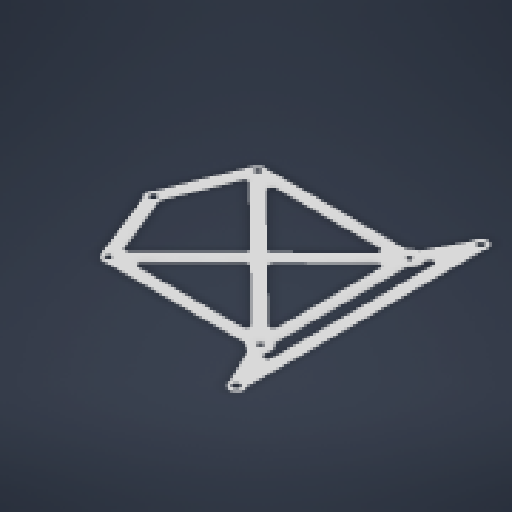
# Autodesk Inventor part: bed
Saved by Autodesk Inventor 2025 (Build 290162000, 162)
## iProperties
Created: 2024-06-24
Part Number: bed
Material: Generic
Document SubType Name: Sheet Metal
Designer: Windows 7 was better
Density: 1 g/cm^3
Sheet Metal Rule: Default_mm
Appearance: Default
Author: Windows 7 was better
Autodesk Inventor part; units mm, degrees
ref_plane "YZ Plane" through (0, 0, 0) normal (1, 0, 0) x (0, 1, 0)
ref_plane "XZ Plane" through (0, 0, 0) normal (0, 1, 0) x (-1, 0, 0)
ref_plane "XY Plane" through (0, 0, 0) normal (0, 0, 1) x (1, 0, 0)
sketch "Sketch1" plane through (0, 0, 0) normal (0, 1, 0) x (-1, 0, 0)
  circle A0 centre (28.351, -169.2998) radius 2.413
  circle A1 centre (28.351, -43.2998) radius 2.413
  circle A2 centre (156.351, -169.2998) radius 2.413
  circle A3 centre (156.351, -43.2998) radius 2.413
  circle A4 centre (8.351, -209.2998) radius 3
  circle A5 centre (8.351, -3.2998) radius 3
  circle A6 centre (181.351, -106.2998) radius 3
  line L0 (16.351, -222.7998) -> (16.351, 9.2002)
  line L1 (8.351, -3.2998) -> (8.351, -209.2998) construction
  line L2 (8.351, -209.2998) -> (181.351, -106.2998) construction
  line L3 (156.351, -43.2998) -> (156.351, -169.2998) construction
  line L4 (156.351, -169.2998) -> (28.351, -169.2998) construction
  line L5 (28.351, -169.2998) -> (28.351, -43.2998) construction
  line L6 (8.351, -106.2998) -> (28.351, -106.2998) construction
  line L7 (8.351, -3.2998) -> (28.351, -43.2998) construction
  line L8 (28.351, -169.2998) -> (8.351, -209.2998) construction
  line L9 (156.351, -43.2998) -> (28.351, -43.2998) construction
  circle A7 centre (156.351, -43.2998) radius 5
  circle A8 centre (156.351, -169.2998) radius 5
  circle A9 centre (8.351, -3.2998) radius 6
  circle A10 centre (8.351, -209.2998) radius 6
  circle A11 centre (181.351, -106.2998) radius 6
  line L10 (156.351, -43.2998) -> (181.351, -106.2998) construction
  line L11 (181.351, -106.2998) -> (156.351, -169.2998) construction
  line L12 (156.351, -43.2998) -> (28.351, -169.2998) construction
  line L13 (28.351, -43.2998) -> (156.351, -169.2998) construction
  line L14 (31.8586, -39.7365) -> (159.8586, -165.7365)
  line L15 (159.8586, -165.7365) -> (152.8434, -172.863)
  line L16 (152.8434, -172.863) -> (24.8434, -46.863)
  line L17 (24.8434, -46.863) -> (31.8586, -39.7365)
  line L18 (31.8586, -39.7365) -> (152.8434, -172.863) construction
  line L19 (159.8586, -165.7365) -> (24.8434, -46.863) construction
  line L20 (152.8434, -39.7365) -> (24.8434, -165.7365)
  line L21 (24.8434, -165.7365) -> (31.8586, -172.863)
  line L22 (31.8586, -172.863) -> (159.8586, -46.863)
  line L23 (159.8586, -46.863) -> (152.8434, -39.7365)
  line L24 (152.8434, -39.7365) -> (31.8586, -172.863) construction
  line L25 (24.8434, -165.7365) -> (159.8586, -46.863) construction
  line L26 (33.351, -43.2998) -> (33.351, -169.2998)
  line L27 (33.351, -169.2998) -> (23.351, -169.2998)
  line L28 (23.351, -169.2998) -> (23.351, -43.2998)
  line L29 (23.351, -43.2998) -> (33.351, -43.2998)
  line L30 (33.351, -43.2998) -> (23.351, -169.2998) construction
  line L31 (33.351, -169.2998) -> (23.351, -43.2998) construction
  line L32 (13.351, -209.2998) -> (13.351, -3.2998)
  line L33 (13.351, -3.2998) -> (3.351, -3.2998)
  line L34 (3.351, -3.2998) -> (3.351, -209.2998)
  line L35 (3.351, -209.2998) -> (13.351, -209.2998)
  line L36 (13.351, -209.2998) -> (3.351, -3.2998) construction
  line L37 (13.351, -3.2998) -> (3.351, -209.2998) construction
  line L38 (3.8789, -5.5359) -> (23.8789, -45.5359)
  line L39 (23.8789, -45.5359) -> (32.8231, -41.0637)
  line L40 (32.8231, -41.0637) -> (12.8231, -1.0637)
  line L41 (12.8231, -1.0637) -> (3.8789, -5.5359)
  line L42 (3.8789, -5.5359) -> (32.8231, -41.0637) construction
  line L43 (23.8789, -45.5359) -> (12.8231, -1.0637) construction
  line L44 (12.8231, -211.5359) -> (32.8231, -171.5359)
  line L45 (32.8231, -171.5359) -> (23.8789, -167.0637)
  line L46 (23.8789, -167.0637) -> (3.8789, -207.0637)
  line L47 (3.8789, -207.0637) -> (12.8231, -211.5359)
  line L48 (12.8231, -211.5359) -> (23.8789, -167.0637) construction
  line L49 (32.8231, -171.5359) -> (3.8789, -207.0637) construction
  line L50 (28.351, -48.2998) -> (156.351, -48.2998)
  line L51 (156.351, -48.2998) -> (156.351, -38.2998)
  line L52 (156.351, -38.2998) -> (28.351, -38.2998)
  line L53 (28.351, -38.2998) -> (28.351, -48.2998)
  line L54 (28.351, -48.2998) -> (156.351, -38.2998) construction
  line L55 (156.351, -48.2998) -> (28.351, -38.2998) construction
  line L56 (28.351, -174.2998) -> (156.351, -174.2998)
  line L57 (156.351, -174.2998) -> (156.351, -164.2998)
  line L58 (156.351, -164.2998) -> (28.351, -164.2998)
  line L59 (28.351, -164.2998) -> (28.351, -174.2998)
  line L60 (28.351, -174.2998) -> (156.351, -164.2998) construction
  line L61 (156.351, -174.2998) -> (28.351, -164.2998) construction
  line L62 (160.9984, -171.144) -> (185.9984, -108.144)
  line L63 (185.9984, -108.144) -> (176.7035, -104.4556)
  line L64 (176.7035, -104.4556) -> (151.7035, -167.4556)
  line L65 (151.7035, -167.4556) -> (160.9984, -171.144)
  line L66 (160.9984, -171.144) -> (176.7035, -104.4556) construction
  line L67 (185.9984, -108.144) -> (151.7035, -167.4556) construction
  line L68 (151.7035, -45.144) -> (176.7035, -108.144)
  line L69 (176.7035, -108.144) -> (185.9984, -104.4556)
  line L70 (185.9984, -104.4556) -> (160.9984, -41.4556)
  line L71 (160.9984, -41.4556) -> (151.7035, -45.144)
  line L72 (151.7035, -45.144) -> (185.9984, -104.4556) construction
  line L73 (176.7035, -108.144) -> (160.9984, -41.4556) construction
  circle A12 centre (28.351, -169.2998) radius 9
  circle A13 centre (28.351, -43.2998) radius 9
  point P0 (0, 0)
  point P1 (92.351, -106.2998)
  point P2 (92.351, -106.2998)
  point P3 (18.351, -23.2998)
  point P4 (18.351, -189.2998)
  point P5 (92.351, -43.2998)
  point P6 (92.351, -169.2998)
  point P7 (168.851, -137.7998)
  point P8 (168.851, -74.7998)
  point P9 (92.351, -99.2837)
  point P10 (40.5578, -48.2998)
  point P11 (144.1442, -48.2998)
  point P12 (13.351, -24.4801)
  point P13 (23.351, -44.4801)
  point P14 (23.351, -168.1194)
  point P15 (13.351, -188.1194)
  point P16 (40.5578, -164.2998)
  point P17 (92.351, -113.3158)
  point P18 (144.1442, -164.2998)
  point P19 (154.4848, -160.4467)
  point P20 (99.4784, -106.2998)
  point P21 (154.4848, -52.1528)
  point P22 (175.4802, -105.0612)
  point P23 (175.4802, -107.5383)
  point P24 (3.351, -6.6164)
  point P25 (3.351, -205.9832)
  point P26 (14.3064, -208.5694)
  point P27 (31.4412, -174.2998)
  point P28 (184.7751, -111.2268)
  point P29 (184.7751, -101.3728)
  point P30 (31.4412, -38.2998)
  point P31 (14.3064, -4.0302)
  point P32 (85.2236, -106.2998)
  point P33 (33.351, -157.3619)
  point P34 (33.351, -55.2377)
  point P35 (20.5322, -38.8426)
  point P36 (23.351, -50.7831)
  point P37 (23.351, -161.8165)
  point P38 (20.5322, -173.757)
  point P39 (29.4765, -178.2291)
  point P40 (35.8343, -174.2998)
  point P41 (35.8343, -38.2998)
  point P42 (29.4765, -34.3704)
  dimension "d11" = 6
  dimension "d12" = 6
  dimension "d39" = 20
  dimension "d40" = 10
  dimension "d41" = 10
  dimension "d44" = 12
  dimension "d45" = 12
  dimension "d46" = 12
  dimension "d47" = 10
  dimension "d48" = 10
  dimension "d49" = 10
  dimension "d50" = 10
  dimension "d51" = 10
  dimension "d52" = 10
  dimension "d53" = 10
  dimension "d54" = 10
  dimension "d55" = 10
  dimension "d56" = 10
  dimension "d58" = 18
  dimension "d59" = 18
  measures "d11" diameter of A4
  measures "d12" diameter of A5
  measures "d39" distance of L6.start L6.end
  measures "d40" diameter of A7
  measures "d41" diameter of A8
  measures "d44" diameter of A9
  measures "d45" diameter of A10
  measures "d46" diameter of A11
  measures "d47" distance of L14.end L15.end
  measures "d48" distance of L21.end L20.end
  measures "d49" distance of L26.end L27.end
  measures "d50" distance of L33.end L32.end
  measures "d51" distance of L39.end L38.end
  measures "d52" distance of L45.end L44.end
  measures "d53" distance of L51.end L50.end
  measures "d54" distance of L57.end L56.end
  measures "d55" distance of L63.end L62.end
  measures "d56" distance of L69.end L68.end
  measures "d58" diameter of A12
  measures "d59" diameter of A13
extrude "Plate1" add sketch "Sketch1" along normal blind 0.5 contours L27 L26 L58 A12 L22 L44 L45 A0 | A0 L59 L58 L26 L27 | A0 L21 L20 A12 L26 L58 L59 | L45 L44 L22 L21 A0 | A0 L45 L46 L28 A12 L20 L21 | L21 L22 L44 L56 L59 A0 | L26 A12 L58 | L27 L28 L46 L45 A0 | A0 L59 L56 L44 A12 L46 L28 L27 | L22 A12 L56 L44 | A12 L20 L26 | L26 L20 L16 L22 L58 A12 | L58 L22 A12 | A12 L28 A13 L16 L26 L20 | L22 L58 L16 A8 L56 A12 | L56 A12 L44 | L46 A12 L28 | L44 L0 L46 A12 | L20 L14 L22 L16 | L16 L26 A13 L50 L14 L20 | L16 A13 L26 | L22 L14 L64 L58 L16 | L58 L64 A8 L16 | A13 L38 L28 | L28 L38 L39 A1 L17 L16 A13 | L44 A10 L32 L46 L0 | L57 A2 L65 A8 | A8 L15 A2 L57 | L20 L50 L68 L22 L14 | L16 L17 A1 L53 L50 L26 A13 | L26 L50 A13 | A8 L65 A2 L15 | L64 L14 A8 L58 | L58 A8 L64 | L38 A13 L40 L52 L53 A1 L29 L28 | L28 L29 A1 L39 L38 | L38 L0 L40 A13 | L44 L47 A4 L35 L32 A10 | A10 L34 L35 A4 L47 L44 | L65 A2 L15 A8 | A8 L14 L64 A11 L62 | L50 A13 L14 | L14 A13 L52 A7 L20 L50 | L20 A7 L68 L50 | L50 L53 A1 L29 L26 | L26 L29 A1 L39 L40 L14 A13 L50 | L68 L50 A7 L22 | L22 A7 L70 A11 L68 | A8 L57 A2 L65 | A8 L15 A2 L57 | L38 L32 A9 L40 L0 | L46 A10 L34 A9 L38 L32 | L32 A10 L46 | A13 L52 L40 | L32 L35 A4 L47 L46 A10 | L62 L63 A6 L69 L70 A11 | A11 L64 L68 L69 A6 L63 L62 | L14 L40 L52 A13 | L23 A3 L71 A7 | A7 L51 A3 L23 | L68 A7 L50 | A11 L68 L64 | L23 A3 L71 A7 | A7 L51 A3 L23 | A11 L70 L69 A6 L63 L64 L68 | L38 A9 L32 | L46 L47 A4 L35 L34 A10 | L40 L14 L17 A1 L53 L52 | L40 L39 A1 L17 L14 | A7 L71 A3 L51 | L71 A3 L51 A7 | L64 L63 A6 L69 L68 | L40 L41 A5 L33 L34 A9 | A9 L32 L33 A5 L41 L40 | A9 L38 L41 A5 L33 L32 | A9 L34 L33 A5 L41 L38
fillet "Corner Round2" radius 3.175 30 edges at (-154.4848, 0.25, -52.1528) (-175.4802, 0.25, -105.0612) (-175.4802, 0.25, -107.5383) (-154.4848, 0.25, -160.4467) (-99.4784, 0.25, -106.2998) (-40.5578, 0.25, -164.2998) (-92.351, 0.25, -113.3158) (-144.1442, 0.25, -164.2998) (-33.351, 0.25, -55.2377) (-85.2236, 0.25, -106.2998) (-33.351, 0.25, -157.3619) (-144.1442, 0.25, -48.2998) (-92.351, 0.25, -99.2837) (-40.5578, 0.25, -48.2998) (-23.351, 0.25, -50.7831) (-23.351, 0.25, -161.8165) (-20.5322, 0.25, -173.757) (-13.351, 0.25, -188.1194) (-13.351, 0.25, -24.4801) (-20.5322, 0.25, -38.8426) (-3.351, 0.25, -6.6164) (-3.351, 0.25, -205.9832) (-14.3064, 0.25, -4.0302) (-29.4765, 0.25, -34.3704) (-35.8343, 0.25, -38.2998) (-184.7751, 0.25, -101.3728) (-184.7751, 0.25, -111.2268) (-35.8343, 0.25, -174.2998) (-29.4765, 0.25, -178.2291) (-14.3064, 0.25, -208.5694)
equation "\"d38\" = Thickness"
equation "\"BendRadius\" = Thickness"
equation "\"BendReliefWidth\" = Thickness"
equation "\"BendReliefDepth\" = 0.5 * Thickness"
equation "\"CornerReliefSize\" = 4 * Thickness"
equation "\"MinimumRemnant\" = 2 * Thickness"
equation "\"TransitionRadius\" = BendRadius"
equation "\"JacobiRadiusSize\" = BendRadius"
equation "\"GapSize\" = Thickness"
equation "\"Thickness\" = 0.5"
body "Solid1"
